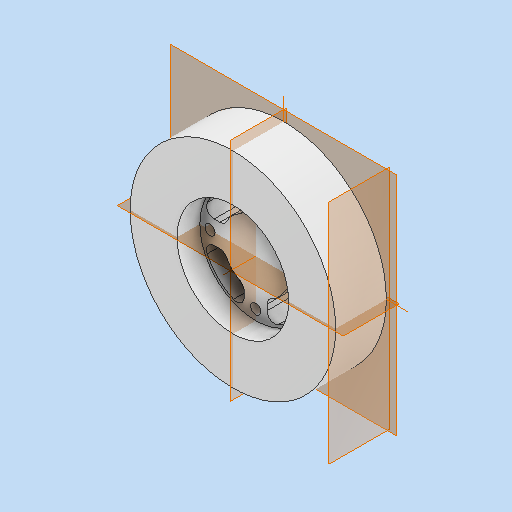
# Autodesk Inventor part: MotorHousing
Saved by Autodesk Inventor 2027 (Build 310192060, 192F)
## iProperties
Created: 2025-04-12
Part Number: MotorHousing
Material: Plastic, Opaque White
Document SubType Name: Modeling
Designer: georg
Density: 0.952 g/cm^3
Appearance: Smooth - White
Mass: 87.7582 g
Surface Area: 190.341 cm^2
Volume: 92.183 cm^3
Author: georg
Autodesk Inventor part; units mm, degrees
sketch "Sketch1" plane through (0, 0, 0) normal (0, 0, 1) x (1, 0, 0)
  circle A0 centre (0, 0) radius 40.5
  dimension "d0" = 81
  constraints: 1 centre point, 1 coincident
  measures "d0" diameter of A0
extrude "Extrusion1" add sketch "Sketch1" along normal blind 20
sketch "Sketch2" plane through (0, 0, 20) normal (0, 0, 1) x (1, 0, 0)
  circle A0 centre (0, 0) radius 22
  dimension "d3" = 44
  constraints: 1 centre point, 1 coincident
  measures "d3" diameter of A0
extrude "Extrusion2" cut sketch "Sketch2" against normal blind 9
sketch "Sketch3" plane through (0, 0, 11) normal (0, 0, 1) x (1, 0, 0)
  circle A0 centre (0, 18) radius 2
  circle A1 centre (-18, 0) radius 2
  circle A2 centre (0, -18) radius 2
  circle A3 centre (18, 0) radius 2
  point P0 (0, 0)
  dimension "d6" = 4
  dimension "d7" = 18
  dimension "d10" = 360
  constraints: 4 centre point, 9 other
  measures "d6" diameter of A0
  measures "d7" distance of point (0, 0) A0.centre
extrude "Extrusion3" cut sketch "Sketch3" against normal blind 12.75
sketch "Sketch4" plane through (0, 0, 11) normal (0, 0, 1) x (1, 0, 0)
  arc A0 (-4.5165, 17.448) -> (-8.8542, 19.2414) centre (-7.5165, 16.3345) ccw
  arc A1 (-8.8542, 19.2414) -> (-19.0977, 9.16) centre (0, 0) ccw
  arc A2 (-14.1333, 4.5) -> (-11.4833, 6.0938) centre (-14.1333, 7.5) ccw
  line L0 (-4.5, 14.1333) -> (-4.5, 16.3631)
  arc A3 (-4.5, 16.3631) -> (-8.75, 19.0902) centre (-7.5, 16.3631) ccw
  arc A4 (-6.0938, 11.4833) -> (-4.5, 14.1333) centre (-7.5, 14.1333) ccw
  arc A5 (-6.0938, 11.4833) -> (-11.4833, 6.0938) centre (0, 0) ccw
  arc A6 (-8.8542, 19.2414) -> (-19.2547, 8.8254) centre (0, 0) ccw
  arc A7 (-8.75, 19.0902) -> (-19.0902, 8.75) centre (0, 0) ccw
  arc A8 (-19.0902, 8.75) -> (-16.3631, 4.5) centre (-16.3631, 7.5) ccw
  line L1 (-16.3631, 4.5) -> (-14.1333, 4.5)
  arc A9 (-11.4833, -6.0938) -> (-14.1333, -4.5) centre (-14.1333, -7.5) ccw
  arc A10 (-4.5, -14.1333) -> (-6.0938, -11.4833) centre (-7.5, -14.1333) ccw
  arc A11 (-11.4833, -6.0938) -> (-6.0938, -11.4833) centre (0, 0) ccw
  line L2 (-14.1333, -4.5) -> (-16.3631, -4.5)
  line L3 (-4.5, -16.3631) -> (-4.5, -14.1333)
  arc A12 (-16.3631, -4.5) -> (-19.0902, -8.75) centre (-16.3631, -7.5) ccw
  arc A13 (-17.448, -4.5165) -> (-19.2414, -8.8542) centre (-16.3345, -7.5165) ccw
  arc A14 (-8.75, -19.0902) -> (-4.5, -16.3631) centre (-7.5, -16.3631) ccw
  arc A15 (-19.0902, -8.75) -> (-8.75, -19.0902) centre (0, 0) ccw
  arc A16 (-19.2414, -8.8542) -> (-9.16, -19.0977) centre (0, 0) ccw
  arc A17 (-19.2414, -8.8542) -> (-8.8254, -19.2547) centre (0, 0) ccw
  arc A18 (6.0938, -11.4833) -> (4.5, -14.1333) centre (7.5, -14.1333) ccw
  arc A19 (14.1333, -4.5) -> (11.4833, -6.0938) centre (14.1333, -7.5) ccw
  arc A20 (6.0938, -11.4833) -> (11.4833, -6.0938) centre (0, 0) ccw
  line L4 (4.5, -14.1333) -> (4.5, -16.3631)
  line L5 (16.3631, -4.5) -> (14.1333, -4.5)
  arc A21 (4.5, -16.3631) -> (8.75, -19.0902) centre (7.5, -16.3631) ccw
  arc A22 (4.5165, -17.448) -> (8.8542, -19.2414) centre (7.5165, -16.3345) ccw
  arc A23 (19.0902, -8.75) -> (16.3631, -4.5) centre (16.3631, -7.5) ccw
  arc A24 (8.75, -19.0902) -> (19.0902, -8.75) centre (0, 0) ccw
  arc A25 (8.8542, -19.2414) -> (19.0977, -9.16) centre (0, 0) ccw
  arc A26 (8.8542, -19.2414) -> (19.2547, -8.8254) centre (0, 0) ccw
  arc A27 (11.4833, 6.0938) -> (14.1333, 4.5) centre (14.1333, 7.5) ccw
  arc A28 (4.5, 14.1333) -> (6.0938, 11.4833) centre (7.5, 14.1333) ccw
  arc A29 (11.4833, 6.0938) -> (6.0938, 11.4833) centre (0, 0) ccw
  line L6 (14.1333, 4.5) -> (16.3631, 4.5)
  line L7 (4.5, 16.3631) -> (4.5, 14.1333)
  arc A30 (16.3631, 4.5) -> (19.0902, 8.75) centre (16.3631, 7.5) ccw
  arc A31 (17.448, 4.5165) -> (19.2414, 8.8542) centre (16.3345, 7.5165) ccw
  arc A32 (8.75, 19.0902) -> (4.5, 16.3631) centre (7.5, 16.3631) ccw
  arc A33 (19.0902, 8.75) -> (8.75, 19.0902) centre (0, 0) ccw
  arc A34 (19.2414, 8.8542) -> (9.16, 19.0977) centre (0, 0) ccw
  arc A35 (19.2414, 8.8542) -> (8.8254, 19.2547) centre (0, 0) ccw
  point P0 (41.0732, 32.7294)
  point P1 (-17.4931, 4.4714)
  point P2 (-16.3796, 7.4714)
  point P3 (-7.4714, -16.3796)
  point P4 (-4.4714, -17.4931)
  point P5 (16.3796, -7.4714)
  point P6 (17.4931, -4.4714)
  point P7 (7.4714, 16.3796)
  point P8 (4.4714, 17.4931)
  dimension "d16" = 360
  constraints: 72 point on circle, 36 centre point, 16 end point, 6 coincident, 157 other
extrude "Extrusion4" cut sketch "Sketch4" against normal blind 12.75
ref_plane "Work Plane1" through (40.7, 0, 0) normal (1, 0, 0) x (0, 1, 0)
body "Solid1"
